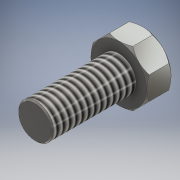
# Autodesk Inventor part: M2.5 6mm screw
Saved by Autodesk Inventor 2016 (Build 200138000, 138)
## iProperties
Created: 2016-07-05
Part Number: M2.5 6mm screw
Material: Steel, High Strength, Low Alloy
Document SubType Name: Modeling
Designer: Jonathan
Density: 7.85 g/cm^3
Appearance: Steel - Polished
Author: Jonathan
Autodesk Inventor part; units mm, degrees
ref_plane "YZ Plane" through (0, 0, 0) normal (1, 0, 0) x (0, 1, 0)
ref_plane "XZ Plane" through (0, 0, 0) normal (0, 1, 0) x (-1, 0, 0)
ref_plane "XY Plane" through (0, 0, 0) normal (0, 0, 1) x (1, 0, 0)
sketch "Sketch1" plane through (0, 0, 0) normal (0, 1, 0) x (-1, 0, 0)
  line L0 (2, 0.8284) -> (2, -0.8284)
  line L1 (2, -0.8284) -> (0.8284, -2)
  line L2 (0.8284, -2) -> (-0.8284, -2)
  line L3 (-0.8284, -2) -> (-2, -0.8284)
  line L4 (-2, -0.8284) -> (-2, 0.8284)
  line L5 (-2, 0.8284) -> (-0.8284, 2)
  line L6 (-0.8284, 2) -> (0.8284, 2)
  line L7 (0.8284, 2) -> (2, 0.8284)
  point P0 (0, 0)
  point P1 (0, -2)
  point P2 (2, 0)
  dimension "d0" = 135
  dimension "d1" = 4
  constraints: 16 end point, 7 equal length, 2 midpoint, 2 parallel, 2 perpendicular, 1 horizontal alignment, 1 vertical, 1 vertical alignment
  measures "d0" angle of L7 L0
  measures "d1" distance between parallel lines of L4 L0
extrude "Extrusion1" add sketch "Sketch1" along normal mid plane 1.75
sketch "Sketch2" plane through (0, 0.875, 0) normal (0, 1, 0) x (1, 0, 0)
  circle A0 centre (0, 0) radius 1.25
  dimension "d4" = 2.5
  constraints: 1 centre point, 1 coincident
  measures "d4" diameter of A0
extrude "Extrusion2" cut sketch "Sketch2" against normal blind 1
thread "Thread1" size "M2.5x0.45" class "6H" standard "ANSI Metric M Profile" full length
chamfer "Chamfer1" distance 0.1 angle 45 1 edges at (-1.25, 0.875, 0)
ref_plane "Work Plane1" through (-0.8284, 0.875, 2) normal (0.9238795, 0, 0.3826834) x (0, -1, 0)
sketch "Sketch3" plane through (-0.8284, 0.875, 2) normal (0.9238795, 0, 0.3826834) x (0, -1, 0)
  line L0 (0, 0) -> (1.75, 0) projected
  line L1 (0, 0) -> (0, 0.6341) projected
  line L2 (0.1768, 0) -> (0, 0.1768)
  line L3 (2.1, 2.1648) -> (-0.35, 2.1648) projected
  point P0 (0.875, 2.1648)
  dimension "d12" = 45
  dimension "d13" = 0.25
  constraints: 2 end point, 2 point on line
  measures "d12" angle of L0 L2
  measures "d13" distance of L2.start L2.end
revolve "Revolution1" cut sketch "Sketch3" angle 360 about axis through (0, -10, 0) along (0, 1, 0)
mirror "Mirror1" about plane through (0, 0, 0) normal (0, 1, 0) of "Revolution1"
sketch "Sketch4" plane through (0, -0.875, 0) normal (0, -1, 0) x (1, 0, 0)
  circle A0 centre (0, 0) radius 1.25
  dimension "d15" = 2.5
  constraints: 1 centre point, 1 coincident
  measures "d15" diameter of A0
extrude "Extrusion3" add sketch "Sketch4" along normal blind 6
chamfer "Chamfer2" distance 0.1 angle 45 1 edges at (-1.25, -6.875, 0)
thread "Thread2" size "M2.5x0.45" class "6g" standard "ANSI Metric M Profile" full length
body "Solid1"
